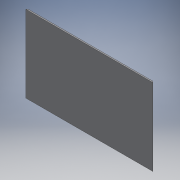
# Autodesk Inventor part: Zwischenplatt
Saved by Autodesk Inventor 2016 SP2 (Build 200236200, 236)
## iProperties
Created: 2018-06-21
Part Number: Zwischenplatt
Material: Generisch
Document SubType Name: Modeling
Designer: Nils
Density: 1 g/cm^3
Appearance: Vorgabe
Author: Nils
Autodesk Inventor part; units mm, degrees
ref_plane "YZ Plane" through (0, 0, 0) normal (1, 0, 0) x (0, 1, 0)
ref_plane "XZ Plane" through (0, 0, 0) normal (0, 1, 0) x (-1, 0, 0)
ref_plane "XY Plane" through (0, 0, 0) normal (0, 0, 1) x (1, 0, 0)
sketch "Skizze1" plane through (0, 0, 0) normal (0, 0, 1) x (1, 0, 0)
  line L0 (153.5, 0) -> (152, 1.5) projected
  line L1 (0, 0) -> (153.5, 0)
  line L2 (152, 1.5) -> (1.5, 1.5)
  line L3 (1.5, 1.5) -> (0, 0)
  dimension "d0" = 45
  constraints: 6 end point, 2 horizontal
  measures "d0" angle of L3 L1
extrude "Extrusion1" add sketch "Skizze1" against normal blind 93
chamfer "Fase1" distance 1.5 angle 45 1 edges at (76.75, 1.5, -93)
